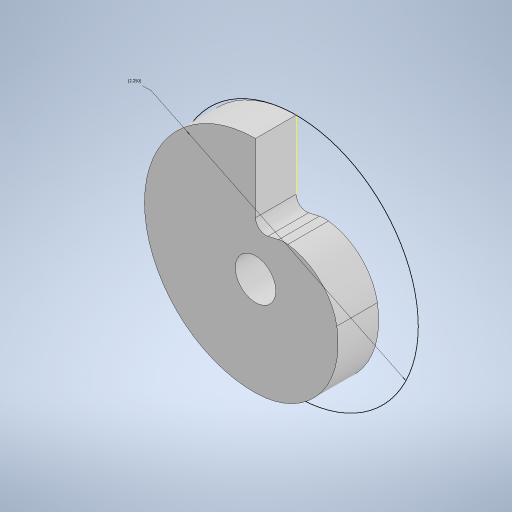
# Autodesk Inventor part: Snail Cam
Saved by Autodesk Inventor 2023.2 (Build 272271000, 271)
## iProperties
Created: 2023-07-06
Part Number: Snail Cam
Material: Generic
Document SubType Name: Modeling
Designer: Nathan Cai
Density: 1 g/cm^3
Appearance: Default
Author: Nathan Cai
Autodesk Inventor part; units mm, degrees
ref_plane "YZ Plane" through (0, 0, 0) normal (1, 0, 0) x (0, 1, 0)
ref_plane "XZ Plane" through (0, 0, 0) normal (0, 1, 0) x (-1, 0, 0)
ref_plane "XY Plane" through (0, 0, 0) normal (0, 0, 1) x (1, 0, 0)
sketch "Sketch1" plane through (0, 0, 0) normal (1, 0, 0) x (0, 1, 0)
  circle A0 centre (0, 0) radius 9.525
  circle A1 centre (0, 0) radius 28.575
  circle A2 centre (0, 0) radius 4.7625
  circle A3 centre (15.875, 41.275) radius 4.7625
  line L0 (15.875, 41.275) -> (27.6665, 7.4435)
  line L1 (-19.9525, 92.075) -> (-19.9525, 41.275)
  circle A4 centre (15.875, 41.275) radius 35.8275
  line L2 (15.875, 41.275) -> (6.87, 6.5977)
  line L3 (0, 0) -> (0, 75.4256) construction
  line L4 (15.875, 41.275) -> (-18.4298, 139.7)
  line L5 (-26.3025, 92.075) -> (-26.3025, 41.275)
  line L6 (-26.3025, 41.275) -> (-13.6025, 41.275)
  line L7 (-13.6025, 41.275) -> (-13.6025, 92.075)
  line L8 (-13.6025, 92.075) -> (-26.3025, 92.075)
  line L9 (-26.3025, 92.075) -> (-13.6025, 41.275) construction
  line L10 (-26.3025, 41.275) -> (-13.6025, 92.075) construction
  point P0 (-19.9525, 66.675)
  dimension "d0" = 19.05
  dimension "d1" = 19.05
  dimension "d2" = 9.525
  dimension "d3" = 9.525
  dimension "d4" = 15.875
  dimension "d5" = 41.275
  dimension "d6" = 33.772
  dimension "d7" = 50.8
  dimension "d8" = 139.7
  dimension "d9" = 12.7
  constraints: 22 end point, 4 centre point, 4 midpoint, 4 parallel, 3 coincident, 3 point on circle, 2 tangent, 1 collinear, 1 perpendicular, 1 vertical, 3 other
  measures "d2" diameter of A2
  measures "d3" diameter of A3
  measures "d4" horizontal distance of A2.centre L0.start
  measures "d5" vertical distance of L0.start point (0, 0)
  measures "d6" angle of L2 L0
  measures "d7" vertical distance of L0.start L1.start
  measures "d8" vertical distance of L3.start L4.end
  measures "d9" distance of L6.end L5.end
sketch "Sketch4" plane through (0, 0, 0) normal (0, 0, 1) x (1, 0, 0)
  circle A0 centre (0, 0) radius 9.525
  circle A1 centre (0, 0) radius 4.7625
  circle A2 centre (0, 0) radius 28.575 construction
  line L0 (0, 0) -> (0, 28.575)
  line L1 (0, 0) -> (28.575, 0) construction
  line L2 (0, 0) -> (-28.575, 0) construction
  line L3 (0, 0) -> (0, -28.575) construction
  circle A3 centre (0, 0) radius 19.05 construction
  circle A4 centre (0, 0) radius 23.114 construction
  circle A5 centre (0, 0) radius 25.908 construction
  arc A6 (19.05, 0) -> (0, 9.525) centre (5.9807, -2.3261) ccw
  arc A7 (0, -23.114) -> (19.05, 0) centre (-0.3155, -3.4467) ccw
  arc A8 (-25.908, 0) -> (0, -23.114) centre (-0.411, 2.5022) ccw
  arc A9 (0, 28.575) -> (-25.908, 0) centre (0, 2.5425) ccw
  line L4 (0, 0) -> (9.525, 16.4978) construction
  line L5 (0, 0) -> (19.05, 0) construction
  line L6 (0, 9.525) -> (6.3187, 10.9443)
  dimension "d61" = 19.05
  dimension "d65" = 46.228
  dimension "d66" = 51.816
  dimension "d62" = 9.525
  dimension "d63" = 19.05
  dimension "d64" = 38.1
  dimension "d68" = 30
  constraints: 15 point on circle, 14 end point, 7 centre point, 6 coincident, 6 point on line, 4 tangent, 2 horizontal, 2 vertical alignment, 1 equal length, 1 horizontal alignment, 1 perpendicular, 1 vertical, 6 other
  measures "d62" diameter of A1
  measures "d64" diameter of A3
  measures "d68" angle of L0 L4
extrude "Extrusion3" add sketch "Sketch4" along normal blind 9.525 contours A0 | L6 A6 A7 A8 A9 L0
fillet "Fillet1" radius 6.35 1 edges at (6.3187, 10.9443, 4.7625)
fillet "Fillet2" radius 2.3813 1 edges at (0, 9.525, 4.7625)
sketch "Sketch5" plane through (0, 0, 0) normal (0, 0, -1) x (-1, 0, 0)
  line L0 (0, 12.5005) -> (0, 28.575) projected
  circle A0 centre (0, 0) radius 28.575
  dimension "d73" = 57.15
  constraints: 1 coincident, 1 vertical alignment, 2 other
body "Solid2"
